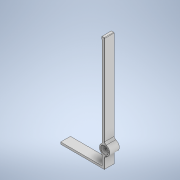
# Autodesk Inventor part: Fan PDP Lid
Saved by Autodesk Inventor 2020.3 (Build 243373010, 373A)
## iProperties
Created: 2019-12-31
Part Number: Fan PDP Lid
Material: Generic
Document SubType Name: Modeling
Designer: pepd9
Density: 1 g/cm^3
Appearance: Default
Author: pepd9
Autodesk Inventor part; units mm, degrees
ref_plane "YZ Plane" through (0, 0, 0) normal (1, 0, 0) x (0, 1, 0)
ref_plane "XZ Plane" through (0, 0, 0) normal (0, 1, 0) x (-1, 0, 0)
ref_plane "XY Plane" through (0, 0, 0) normal (0, 0, 1) x (1, 0, 0)
sketch "Sketch1" plane through (0, 0, 0) normal (0, 0, 1) x (1, 0, 0)
  line L0 (17.1597, -40.1235) -> (17.1597, -50)
  line L1 (17.1597, -50) -> (19.1597, -50)
  line L2 (19.1597, -50) -> (19.1597, -41.1847)
  arc A0 (20.5443, -39.2817) -> (19.1597, -41.1847) centre (21.1597, -41.1847) ccw
  arc A1 (20.5443, -39.2817) -> (20.5443, -30.7183) centre (19.1597, -35) ccw
  arc A2 (19.1597, -28.8153) -> (20.5443, -30.7183) centre (21.1597, -28.8153) ccw
  line L3 (19.1597, -28.8153) -> (19.1597, 49.6)
  arc A3 (19.1597, 49.6) -> (18.7597, 50) centre (18.7597, 49.6) ccw
  line L4 (18.7597, 50) -> (16.7597, 50)
  arc A4 (17.1597, 47.6) -> (16.7597, 48) centre (16.7597, 47.6) ccw
  line L5 (17.1597, 47.6) -> (17.1597, -29.8765)
  arc A5 (16.3905, -31.453) -> (17.1597, -29.8765) centre (15.1597, -29.8765) ccw
  arc A6 (16.3905, -31.453) -> (16.3905, -38.547) centre (19.1597, -35) ccw
  arc A7 (17.1597, -40.1235) -> (16.3905, -38.547) centre (15.1597, -40.1235) ccw
  line L6 (-19.1597, -50) -> (19.1597, -50)
  line L7 (19.1597, -50) -> (19.1597, -48)
  line L8 (19.1597, -48) -> (-19.1597, -48)
  line L9 (-19.1597, -48) -> (-19.1597, -50)
  circle A8 centre (19.1597, -35) radius 2.2
  line L10 (16.7597, 50) -> (16.7597, 48)
  point P0 (0, 0)
  point P1 (17.1605, -50)
  point P2 (17.1597, -48)
  dimension "d0" = 2
  constraints: 22 end point, 16 point on circle, 9 centre point, 1 horizontal, 1 parallel, 1 point on line
  measures "d0" distance between parallel lines of L8 L6
extrude "Extrusion1" add sketch "Sketch1" along normal blind 7 contours A7 A6 A5 L5 A4 L10 L4 A3 L3 A2 A1 A0 L2 L8 L0 | L8 L2 L1 L0 | L0 L6 L9 L8 | A8
sketch "Sketch2" plane through (0, 0, 7) normal (0, 0, 1) x (1, 0, 0)
  line L0 (-19.1597, -50) -> (19.1597, -50) projected
  line L1 (19.1597, -50) -> (19.1597, -41.1847) projected
  arc A0 (20.5443, -39.2817) -> (19.1597, -41.1847) centre (21.1597, -41.1847) ccw projected
  arc A1 (20.5443, -39.2817) -> (20.5443, -30.7183) centre (19.1597, -35) ccw projected
  arc A2 (19.1597, -28.8153) -> (20.5443, -30.7183) centre (21.1597, -28.8153) ccw projected
  line L2 (19.1597, -28.8153) -> (19.1597, 49.6) projected
  arc A3 (19.1597, 49.6) -> (18.7597, 50) centre (18.7597, 49.6) ccw projected
  line L3 (18.7597, 50) -> (16.7597, 50) projected
  arc A4 (17.1597, 47.6) -> (16.7597, 48) centre (16.7597, 47.6) ccw projected
  line L4 (17.1597, 47.6) -> (17.1597, -29.8765) projected
  arc A5 (16.3905, -31.453) -> (17.1597, -29.8765) centre (15.1597, -29.8765) ccw projected
  arc A6 (16.3905, -31.453) -> (16.3905, -38.547) centre (19.1597, -35) ccw projected
  arc A7 (17.1597, -40.1235) -> (16.3905, -38.547) centre (15.1597, -40.1235) ccw projected
  line L5 (17.1597, -40.1235) -> (17.1597, -48) projected
  line L6 (17.1597, -48) -> (-19.1597, -48) projected
  line L7 (16.7597, 50) -> (16.7597, 48) projected
  line L8 (-19.1597, -48) -> (-19.1597, -50) projected
  point P0 (0, 0)
extrude "Extrusion2" add sketch "Sketch2" along normal blind 1.5
fillet "Fillet1" radius 0.4 2 edges at (19.1597, -50, 7.75) (19.1597, -50, 3.5)
sketch "Sketch3" plane through (0, 0, 8.5) normal (0, 0, 1) x (1, 0, 0)
  line L0 (-17.1597, -48) -> (-17.1597, 26.9323) projected
  line L1 (-19.1597, -50) -> (18.7597, -50) projected
  arc A0 (18.7597, -50) -> (19.1597, -49.6) centre (18.7597, -49.6) ccw projected
  line L2 (19.1597, -49.6) -> (19.1597, -41.1847) projected
  arc A1 (20.5443, -39.2817) -> (19.1597, -41.1847) centre (21.1597, -41.1847) ccw projected
  arc A2 (20.5443, -39.2817) -> (20.5443, -30.7183) centre (19.1597, -35) ccw projected
  arc A3 (19.1597, -28.8153) -> (20.5443, -30.7183) centre (21.1597, -28.8153) ccw projected
  line L3 (19.1597, -28.8153) -> (19.1597, 49.6) projected
  arc A4 (19.1597, 49.6) -> (18.7597, 50) centre (18.7597, 49.6) ccw projected
  line L4 (18.7597, 50) -> (16.7597, 50) projected
  line L5 (16.7597, 50) -> (16.7597, 48) projected
  arc A5 (17.1597, 47.6) -> (16.7597, 48) centre (16.7597, 47.6) ccw projected
  line L6 (17.1597, 47.6) -> (17.1597, -29.8765) projected
  arc A6 (16.3905, -31.453) -> (17.1597, -29.8765) centre (15.1597, -29.8765) ccw projected
  arc A7 (16.3905, -31.453) -> (16.3905, -38.547) centre (19.1597, -35) ccw projected
  arc A8 (17.1597, -40.1235) -> (16.3905, -38.547) centre (15.1597, -40.1235) ccw projected
  line L7 (17.1597, -40.1235) -> (17.1597, -48) projected
  line L8 (17.1597, -48) -> (-19.1597, -48) projected
  line L9 (-19.1597, -48) -> (-19.1597, -50) projected
  point P0 (0, 0)
  point P1 (-4.5248, -20.5041)
  point P2 (-13.7791, 32.7713)
  constraints: 1 other
hole "Hole1" at (19.1597, -35, 8.5) at (-13.7791, 32.7713, 8.5) direction (0, 0, -1) diameter 3.4 end through all counterbore diameter 6.5 counterbore depth 3 clearance for "Socket Head Cap Screw" size "M3" standard "Ansi Metric M Profile"
sketch "Sketch4" plane through (19.1597, -35, 5.5) normal (0, 0, 1) x (1, 0, 0)
  circle A0 centre (0, 0) radius 3.25 projected
  circle A1 centre (0, 0) radius 3.25 projected
  circle A2 centre (0, 0) radius 1.7 projected
  circle A3 centre (-32.9388, 67.7713) radius 3.25 projected
  circle A4 centre (-32.9388, 67.7713) radius 1.7 projected
  line L0 (6.1601, -1.7) -> (-6.1601, -1.7)
  line L1 (-6.1601, -1.7) -> (-6.1601, 1.7)
  line L2 (-6.1601, 1.7) -> (6.1601, 1.7)
  line L3 (6.1601, 1.7) -> (6.1601, -1.7)
  circle A5 centre (0, 0) radius 3.25 projected
  line L4 (6.1601, -1.7) -> (-6.1601, 1.7) construction
  line L5 (-6.1601, -1.7) -> (6.1601, 1.7) construction
  arc A6 (-35.3905, 72.9289) -> (-38.3194, 65.8579) centre (-28.3194, 65.8579) ccw projected
  line L6 (-28.2339, 66.0713) -> (-37.6437, 66.0713)
  line L7 (-37.6437, 66.0713) -> (-37.6437, 69.4713)
  line L8 (-37.6437, 69.4713) -> (-28.2339, 69.4713)
  line L9 (-28.2339, 69.4713) -> (-28.2339, 66.0713)
  circle A7 centre (-32.9388, 67.7713) radius 1.7 projected
  line L10 (-28.2339, 66.0713) -> (-37.6437, 69.4713) construction
  line L11 (-37.6437, 66.0713) -> (-28.2339, 69.4713) construction
  point P0 (-19.1597, 35)
  point P1 (-30.1689, 69.4713)
  point P2 (-32.9388, 69.4713)
  point P3 (-32.9388, 66.0713)
  point P4 (-30.1689, 66.0713)
  point P5 (-35.7087, 69.4713)
  point P6 (-35.7087, 66.0713)
  point P7 (0, 1.7)
  point P8 (-2.7699, 1.7)
  point P9 (-2.7699, -1.7)
  point P10 (0, -1.7)
  point P11 (2.7699, 1.7)
  point P12 (2.7699, -1.7)
  dimension "d13" = 3.4
  dimension "d14" = 3.4
  constraints: 24 end point, 4 midpoint, 4 parallel, 2 horizontal, 2 perpendicular, 1 point on circle
  measures "d13" distance of L0.end L1.end
  measures "d14" distance of L6.end L7.end
extrude "Extrusion3" cut sketch "Sketch4" against normal blind 0.5 contours A0 L0 A2 L2 | L2 A2 L0 A0 | A3 L6 A4 L8 | L8 A4 L6 A3
sketch "Sketch5" plane through (19.1597, -35, 5) normal (0, 0, 1) x (1, 0, 0)
  arc A0 (-32.9388, 69.4713) -> (-32.9388, 66.0713) centre (-32.9388, 67.7713) ccw projected
  line L0 (-35.7087, 69.4713) -> (-32.9388, 69.4713) projected
  arc A1 (-35.7087, 69.4713) -> (-35.7087, 66.0713) centre (-32.9388, 67.7713) ccw projected
  line L1 (-32.9388, 66.0713) -> (-35.7087, 66.0713) projected
  arc A2 (-30.1689, 66.0713) -> (-30.1689, 69.4713) centre (-32.9388, 67.7713) ccw projected
  line L2 (-32.9388, 69.4713) -> (-30.1689, 69.4713) projected
  arc A3 (-32.9388, 66.0713) -> (-32.9388, 69.4713) centre (-32.9388, 67.7713) ccw projected
  line L3 (-30.1689, 66.0713) -> (-32.9388, 66.0713) projected
  arc A4 (0, 1.7) -> (0, -1.7) centre (0, 0) ccw projected
  line L4 (-2.7699, 1.7) -> (0, 1.7) projected
  arc A5 (-2.7699, 1.7) -> (-2.7699, -1.7) centre (0, 0) ccw projected
  line L5 (0, -1.7) -> (-2.7699, -1.7) projected
  line L6 (2.7699, -1.7) -> (0, -1.7) projected
  arc A6 (2.7699, -1.7) -> (2.7699, 1.7) centre (0, 0) ccw projected
  line L7 (0, 1.7) -> (2.7699, 1.7) projected
  arc A7 (0, -1.7) -> (0, 1.7) centre (0, 0) ccw projected
  line L8 (1.7, 1.7) -> (-1.7, 1.7)
  line L9 (-1.7, 1.7) -> (-1.7, -1.7)
  line L10 (-1.7, -1.7) -> (1.7, -1.7)
  line L11 (1.7, -1.7) -> (1.7, 1.7)
  line L12 (1.7, 1.7) -> (-1.7, -1.7) construction
  line L13 (-1.7, 1.7) -> (1.7, -1.7) construction
  line L14 (-31.2388, 66.0713) -> (-34.6388, 66.0713)
  line L15 (-34.6388, 66.0713) -> (-34.6388, 69.4713)
  line L16 (-34.6388, 69.4713) -> (-31.2388, 69.4713)
  line L17 (-31.2388, 69.4713) -> (-31.2388, 66.0713)
  line L18 (-31.2388, 66.0713) -> (-34.6388, 69.4713) construction
  line L19 (-34.6388, 66.0713) -> (-31.2388, 69.4713) construction
  point P0 (-19.1597, 35)
  point P1 (1.7, -1.7)
  point P2 (1.7, 1.7)
  point P3 (-1.7, 1.7)
  point P4 (-1.7, -1.7)
  dimension "d17" = 3.4
  dimension "d18" = 3.4
  dimension "d19" = 3.4
  dimension "d20" = 3.4
  constraints: 24 end point, 4 midpoint, 4 parallel, 2 horizontal, 2 perpendicular
  measures "d17" distance of L10.end L9.end
  measures "d18" distance of L9.end L8.end
  measures "d19" distance of L15.end L16.end
  measures "d20" distance of L14.end L15.end
extrude "Extrusion4" cut sketch "Sketch5" against normal blind 0.5 contours A3 A0 | A0 L15 L0 | L2 L17 A3 | A0 L1 L15 | L17 L3 A3 | A7 A4 | A4 L9 L4 | L7 L11 A7 | A4 L5 L9 | L11 L6 A7
sketch "Sketch6" plane through (0, 0, 8.5) normal (0, 0, 1) x (1, 0, 0)
  line L0 (-17.2523, -48.0084) -> (-17.2523, -4.1232) construction
  line L1 (-17.2523, -4.1232) -> (-6.8496, -4.1232) construction
  line L2 (-6.8496, -4.1232) -> (-6.8496, -48.0084) construction
  line L3 (-6.8496, -48.0084) -> (-17.2523, -48.0084) construction
  line L4 (-6.9988, -47.4715) -> (-16.9988, -47.4715)
  line L5 (-16.9988, -47.4715) -> (-16.9988, -43.5714)
  spline S0 degree 2 poles (-16.9988, -43.5714) (-16.9988, -42.2142) (-15.8131, -40.8048) (-14.5379, -40.596) knots 0 0 0 1 2 2 2
  spline S1 degree 2 poles (-14.5379, -40.596) (-14.1203, -40.5364) (-13.8295, -40.5214) (-13.7176, -40.5214) knots 0 0 0 1 2 2 2
  spline S2 degree 2 poles (-13.7176, -40.5214) (-12.3082, -40.5214) (-10.7273, -42.2664) (-10.7273, -43.825) knots 0 0 0 1 2 2 2
  line L6 (-10.7273, -43.825) -> (-10.7273, -44.6154)
  line L7 (-10.7273, -44.6154) -> (-6.9988, -44.6154)
  line L8 (-6.9988, -44.6154) -> (-6.9988, -47.4715)
  spline S3 degree 2 poles (-12.8302, -44.1904) (-12.8302, -43.9816) (-13.1807, -43.5341) (-13.5387, -43.4596) knots 0 0 0 1 2 2 2
  spline S4 degree 2 poles (-13.5387, -43.4596) (-13.7251, -43.4223) (-13.8892, -43.4223) knots 0 0 0 1 1 1
  spline S5 degree 2 poles (-13.8892, -43.4223) (-14.3515, -43.4223) (-14.8809, -43.8548) (-14.8809, -44.1605) knots 0 0 0 1 2 2 2
  line L9 (-14.8809, -44.1605) -> (-14.8809, -44.6154)
  line L10 (-14.8809, -44.6154) -> (-12.8302, -44.6154)
  line L11 (-12.8302, -44.6154) -> (-12.8302, -44.1904)
  line L12 (-6.9988, -40.1188) -> (-16.9988, -40.1188)
  line L13 (-16.9988, -40.1188) -> (-16.9988, -34.1083)
  line L14 (-16.9988, -34.1083) -> (-14.6871, -34.1083)
  line L15 (-14.6871, -34.1083) -> (-14.6871, -37.2627)
  line L16 (-14.6871, -37.2627) -> (-13.1956, -37.2627)
  line L17 (-13.1956, -37.2627) -> (-13.1956, -34.3022)
  line L18 (-13.1956, -34.3022) -> (-10.9809, -34.3022)
  line L19 (-10.9809, -34.3022) -> (-10.9809, -37.2627)
  line L20 (-10.9809, -37.2627) -> (-9.3105, -37.2627)
  line L21 (-9.3105, -37.2627) -> (-9.3105, -34.0039)
  line L22 (-9.3105, -34.0039) -> (-6.9988, -34.0039)
  line L23 (-6.9988, -34.0039) -> (-6.9988, -40.1188)
  line L24 (-6.9988, -33.3552) -> (-16.9988, -33.3552)
  line L25 (-16.9988, -33.3552) -> (-16.9988, -29.4551)
  spline S6 degree 2 poles (-16.9988, -29.4551) (-16.9988, -28.0979) (-15.8131, -26.6885) (-14.5379, -26.4797) knots 0 0 0 1 2 2 2
  spline S7 degree 2 poles (-14.5379, -26.4797) (-14.1203, -26.42) (-13.8295, -26.4051) (-13.7176, -26.4051) knots 0 0 0 1 2 2 2
  spline S8 degree 2 poles (-13.7176, -26.4051) (-12.3082, -26.4051) (-10.7273, -28.1501) (-10.7273, -29.7086) knots 0 0 0 1 2 2 2
  line L26 (-10.7273, -29.7086) -> (-10.7273, -30.4991)
  line L27 (-10.7273, -30.4991) -> (-6.9988, -30.4991)
  line L28 (-6.9988, -30.4991) -> (-6.9988, -33.3552)
  spline S9 degree 2 poles (-12.8302, -30.074) (-12.8302, -29.8652) (-13.1807, -29.4178) (-13.5387, -29.3432) knots 0 0 0 1 2 2 2
  spline S10 degree 2 poles (-13.5387, -29.3432) (-13.7251, -29.3059) (-13.8892, -29.3059) knots 0 0 0 1 1 1
  spline S11 degree 2 poles (-13.8892, -29.3059) (-14.3515, -29.3059) (-14.8809, -29.7384) (-14.8809, -30.0442) knots 0 0 0 1 2 2 2
  line L29 (-14.8809, -30.0442) -> (-14.8809, -30.4991)
  line L30 (-14.8809, -30.4991) -> (-12.8302, -30.4991)
  line L31 (-12.8302, -30.4991) -> (-12.8302, -30.074)
  line L32 (-13.2255, -15.3835) -> (-13.2255, -18.1352)
  line L33 (-13.2255, -18.1352) -> (-13.8892, -18.1426)
  spline S12 degree 2 poles (-13.8892, -18.1426) (-14.3813, -18.1426) (-14.7169, -18.1948) (-15.0226, -18.3216) (-15.1718, -18.5751) (-15.1718, -18.7392) knots 0 0 0 1 2 3 4 4 4
  spline S13 degree 2 poles (-15.1718, -18.7392) (-15.1718, -18.9331) (-14.866, -19.2388) (-13.8817, -19.3134) (-11.8235, -19.3134) knots 0 0 0 1 2 3 3 3
  spline S14 degree 2 poles (-11.8235, -19.3134) (-10.2202, -19.3134) (-9.2807, -19.2388) (-9.0868, -19.1419) knots 0 0 0 1 2 2 2
  spline S15 degree 2 poles (-9.0868, -19.1419) (-8.781, -18.9853) (-8.781, -18.6572) knots 0 0 0 1 1 1
  spline S16 degree 2 poles (-8.781, -18.6572) (-8.781, -18.4558) (-9.0868, -18.1501) (-9.7057, -18.0457) (-10.7199, -18.0457) knots 0 0 0 1 2 3 3 3
  line L34 (-10.7199, -18.0457) -> (-11.1673, -18.0457)
  line L35 (-11.1673, -18.0457) -> (-11.1673, -15.2567)
  spline S17 degree 2 poles (-11.1673, -15.2567) (-10.8839, -15.2567) (-10.6006, -15.2567) (-10.4514, -15.2567) knots 0 0 0 1 2 2 2
  spline S18 degree 2 poles (-10.4514, -15.2567) (-8.6319, -15.2567) (-6.8496, -16.9495) (-6.8496, -18.7168) knots 0 0 0 1 2 2 2
  spline S19 degree 2 poles (-6.8496, -18.7168) (-6.8496, -19.0822) (-6.8944, -19.4849) knots 0 0 0 1 1 1
  spline S20 degree 2 poles (-6.8944, -19.4849) (-7.0211, -20.9465) (-8.0204, -21.5654) knots 0 0 0 1 1 1
  spline S21 degree 2 poles (-8.0204, -21.5654) (-9.0495, -22.1993) (-11.391, -22.1993) knots 0 0 0 1 1 1
  line L36 (-11.391, -22.1993) -> (-11.7937, -22.2366)
  line L37 (-11.7937, -22.2366) -> (-11.9876, -22.2366)
  line L38 (-11.9876, -22.2366) -> (-13.5387, -22.1993)
  spline S22 degree 2 poles (-13.5387, -22.1993) (-15.224, -22.1993) (-16.9242, -20.7899) (-17.0883, -19.2985) knots 0 0 0 1 2 2 2
  spline S23 degree 2 poles (-17.0883, -19.2985) (-17.133, -18.8212) (-17.133, -18.4484) knots 0 0 0 1 1 1
  spline S24 degree 2 poles (-17.133, -18.4484) (-17.133, -16.8525) (-15.4328, -15.3835) (-13.6282, -15.3835) knots 0 0 0 1 2 2 2
  line L39 (-13.6282, -15.3835) -> (-13.2255, -15.3835)
  spline S25 degree 2 poles (-12.2038, -14.9286) (-14.3291, -14.9286) (-15.6043, -14.2053) knots 0 0 0 1 1 1
  spline S26 degree 2 poles (-15.6043, -14.2053) (-17.2523, -13.2806) (-17.2523, -11.3194) knots 0 0 0 1 1 1
  spline S27 degree 2 poles (-17.2523, -11.3194) (-17.2523, -10.7079) (-17.0584, -9.895) (-16.872, -9.5669) knots 0 0 0 1 2 2 2
  spline S28 degree 2 poles (-16.872, -9.5669) (-16.35, -8.4931) (-14.4335, -7.7325) (-12.2038, -7.7325) knots 0 0 0 1 2 2 2
  spline S29 degree 2 poles (-12.2038, -7.7325) (-9.3776, -7.7325) (-6.8795, -9.0151) (-6.8795, -10.5438) knots 0 0 0 1 2 2 2
  spline S30 degree 2 poles (-6.8795, -10.5438) (-6.8795, -12.4752) (-7.476, -13.4894) knots 0 0 0 1 1 1
  spline S31 degree 2 poles (-7.476, -13.4894) (-8.0055, -14.3842) (-9.0644, -14.7049) knots 0 0 0 1 1 1
  spline S32 degree 2 poles (-9.0644, -14.7049) (-9.7952, -14.9286) (-11.1748, -14.9286) knots 0 0 0 1 1 1
  spline S33 degree 2 poles (-11.1748, -14.9286) (-11.4208, -14.9286) (-11.9279, -14.9286) (-12.2038, -14.9286) knots 0 0 0 1 2 2 2
  spline S34 degree 2 poles (-11.309, -12.0054) (-9.6908, -12.0054) (-8.7959, -11.7071) (-8.7959, -11.3194) knots 0 0 0 1 2 2 2
  spline S35 degree 2 poles (-8.7959, -11.3194) (-8.7959, -10.954) (-9.6833, -10.6557) (-11.309, -10.6557) knots 0 0 0 1 2 2 2
  line L40 (-11.309, -10.6557) -> (-12.7408, -10.6557)
  spline S36 degree 2 poles (-12.7408, -10.6557) (-14.3217, -10.6557) (-15.2165, -10.954) (-15.2165, -11.3194) knots 0 0 0 1 2 2 2
  spline S37 degree 2 poles (-15.2165, -11.3194) (-15.2165, -11.6922) (-14.3291, -12.0054) (-12.7408, -12.0054) knots 0 0 0 1 2 2 2
  line L41 (-12.7408, -12.0054) -> (-11.309, -12.0054)
  line L42 (-6.9988, -7.0241) -> (-9.6982, -7.0241)
  line L43 (-9.6982, -7.0241) -> (-9.6982, -4.4141)
  line L44 (-9.6982, -4.4141) -> (-6.9988, -4.4141)
  line L45 (-6.9988, -4.4141) -> (-6.9988, -7.0241)
  point P0 (0, 0)
  constraints: 2 other
extrude "Extrusion5" cut sketch "Sketch6" against normal blind 0.6
sketch "Sketch7" plane through (0, 0, 8.5) normal (0, 0, 1) x (1, 0, 0)
  line L0 (-3.7937, -33.6465) -> (-3.7937, -2.887) construction
  line L1 (-3.7937, -2.887) -> (-12.6472, -2.887) construction
  line L2 (-12.6472, -2.887) -> (-12.6472, -33.6465) construction
  line L3 (-12.6472, -33.6465) -> (-3.7937, -33.6465) construction
  line L4 (3.9744, -28.2269) -> (3.9744, 29.3109) construction
  line L5 (3.9744, 29.3109) -> (-4.8792, 29.3109) construction
  line L6 (-4.8792, 29.3109) -> (-4.8792, -28.2269) construction
  line L7 (-4.8792, -28.2269) -> (3.9744, -28.2269) construction
  line L8 (-3.7937, -31.8232) -> (-1.4209, -32.0663)
  line L9 (-1.4209, -32.0663) -> (-1.4209, -32.8929)
  line L10 (-1.4209, -32.8929) -> (-3.7937, -33.136)
  line L11 (-3.7937, -33.136) -> (-3.7937, -31.8232)
  line L12 (-3.7937, -30.1263) -> (-1.4209, -30.3694)
  line L13 (-1.4209, -30.3694) -> (-1.4209, -31.196)
  line L14 (-1.4209, -31.196) -> (-3.7937, -31.4391)
  line L15 (-3.7937, -31.4391) -> (-3.7937, -30.1263)
  line L16 (2.4737, -27.8362) -> (-2.3837, -27.8362)
  line L17 (-2.3837, -27.8362) -> (-2.3837, -29.6109)
  line L18 (-2.3837, -29.6109) -> (-3.5263, -29.6109)
  line L19 (-3.5263, -29.6109) -> (-3.5263, -24.5541)
  line L20 (-3.5263, -24.5541) -> (-2.3837, -24.5541)
  line L21 (-2.3837, -24.5541) -> (-2.3837, -26.3289)
  line L22 (-2.3837, -26.3289) -> (2.4737, -26.3289)
  line L23 (2.4737, -26.3289) -> (2.4737, -27.8362)
  line L24 (2.4737, -23.9366) -> (-3.5263, -23.9366)
  line L25 (-3.5263, -23.9366) -> (-3.5263, -19.8815)
  line L26 (-3.5263, -19.8815) -> (-2.3837, -19.8815)
  line L27 (-2.3837, -19.8815) -> (-2.3837, -22.4391)
  line L28 (-2.3837, -22.4391) -> (-1.3285, -22.4391)
  line L29 (-1.3285, -22.4391) -> (-1.3285, -20.0809)
  line L30 (-1.3285, -20.0809) -> (-0.1859, -20.0809)
  line L31 (-0.1859, -20.0809) -> (-0.1859, -22.4391)
  line L32 (-0.1859, -22.4391) -> (1.3311, -22.4391)
  line L33 (1.3311, -22.4391) -> (1.3311, -19.8815)
  line L34 (1.3311, -19.8815) -> (2.4737, -19.8815)
  line L35 (2.4737, -19.8815) -> (2.4737, -23.9366)
  line L36 (2.4737, -12.734) -> (2.4737, -14.2316)
  line L37 (2.4737, -14.2316) -> (-1.5036, -14.2316)
  line L38 (-1.5036, -14.2316) -> (1.0637, -15.3208)
  line L39 (1.0637, -15.3208) -> (1.0637, -16.3515)
  line L40 (1.0637, -16.3515) -> (-1.5036, -17.4407)
  line L41 (-1.5036, -17.4407) -> (2.4737, -17.4407)
  line L42 (2.4737, -17.4407) -> (2.4737, -18.8605)
  line L43 (2.4737, -18.8605) -> (-3.5263, -18.8605)
  line L44 (-3.5263, -18.8605) -> (-3.5263, -17.1246)
  line L45 (-3.5263, -17.1246) -> (-0.5652, -15.7924)
  line L46 (-0.5652, -15.7924) -> (-3.5263, -14.4699)
  line L47 (-3.5263, -14.4699) -> (-3.5263, -12.734)
  line L48 (-3.5263, -12.734) -> (2.4737, -12.734)
  spline S0 degree 2 poles (-1.6349, -6.875) (-1.2167, -6.875) (-0.4582, -7.1425) (-0.2054, -7.3904) knots 0 0 0 1 2 2 2
  spline S1 degree 2 poles (-0.2054, -7.3904) (-0.0449, -7.5412) (0.2176, -7.9107) (0.31, -8.1295) knots 0 0 0 1 2 2 2
  spline S2 degree 2 poles (0.31, -8.1295) (0.4024, -8.3532) (0.5094, -8.8734) (0.5094, -9.1943) knots 0 0 0 1 2 2 2
  line L49 (0.5094, -9.1943) -> (0.5094, -9.982)
  line L50 (0.5094, -9.982) -> (2.4737, -9.982)
  line L51 (2.4737, -9.982) -> (2.4737, -11.4893)
  line L52 (2.4737, -11.4893) -> (-3.5263, -11.4893)
  line L53 (-3.5263, -11.4893) -> (-3.5263, -9.1603)
  spline S3 degree 2 poles (-3.5263, -9.1603) (-3.5263, -8.6449) (-3.3367, -7.8913) (-3.1324, -7.5849) knots 0 0 0 1 2 2 2
  spline S4 degree 2 poles (-3.1324, -7.5849) (-2.9039, -7.2446) (-2.1551, -6.875) (-1.6349, -6.875) knots 0 0 0 1 2 2 2
  spline S5 degree 2 poles (-1.596, -8.4212) (-1.8537, -8.4212) (-2.2183, -8.6644) (-2.2864, -8.8297) knots 0 0 0 1 2 2 2
  spline S6 degree 2 poles (-2.2864, -8.8297) (-2.3788, -9.0436) (-2.408, -9.4326) (-2.408, -9.7681) knots 0 0 0 1 2 2 2
  line L54 (-2.408, -9.7681) -> (-2.408, -9.982)
  line L55 (-2.408, -9.982) -> (-0.6089, -9.982)
  line L56 (-0.6089, -9.982) -> (-0.6089, -9.875)
  spline S7 degree 2 poles (-0.6089, -9.875) (-0.6089, -9.666) (-0.6187, -9.2867) (-0.643, -9.1457) knots 0 0 0 1 2 2 2
  spline S8 degree 2 poles (-0.643, -9.1457) (-0.6624, -9.0242) (-0.7791, -8.7567) (-0.852, -8.6838) knots 0 0 0 1 2 2 2
  spline S9 degree 2 poles (-0.852, -8.6838) (-0.9979, -8.5282) (-1.3237, -8.4212) (-1.596, -8.4212) knots 0 0 0 1 2 2 2
  spline S10 degree 2 poles (-0.5263, -0.6076) (0.9324, -0.6076) (2.6001, -2.1635) (2.6001, -3.5152) knots 0 0 0 1 2 2 2
  spline S11 degree 2 poles (2.6001, -3.5152) (2.6001, -4.8718) (0.9129, -6.418) (-0.5263, -6.418) knots 0 0 0 1 2 2 2
  spline S12 degree 2 poles (-0.5263, -6.418) (-1.9704, -6.418) (-3.6527, -4.8718) (-3.6527, -3.5152) knots 0 0 0 1 2 2 2
  spline S13 degree 2 poles (-3.6527, -3.5152) (-3.6527, -2.1635) (-1.9801, -0.6076) (-0.5263, -0.6076) knots 0 0 0 1 2 2 2
  spline S14 degree 2 poles (-0.5263, -2.1635) (-1.066, -2.1635) (-1.8196, -2.3823) (-2.0579, -2.572) knots 0 0 0 1 2 2 2
  spline S15 degree 2 poles (-2.0579, -2.572) (-2.3059, -2.7616) (-2.5198, -3.2478) (-2.5198, -3.5104) knots 0 0 0 1 2 2 2
  spline S16 degree 2 poles (-2.5198, -3.5104) (-2.5198, -3.7875) (-2.3204, -4.2397) (-2.0676, -4.4488) knots 0 0 0 1 2 2 2
  spline S17 degree 2 poles (-2.0676, -4.4488) (-1.8342, -4.6336) (-1.0611, -4.8621) (-0.5263, -4.8621) knots 0 0 0 1 2 2 2
  spline S18 degree 2 poles (-0.5263, -4.8621) (0.028, -4.8621) (0.7574, -4.6433) (1.0053, -4.4537) knots 0 0 0 1 2 2 2
  spline S19 degree 2 poles (1.0053, -4.4537) (1.2533, -4.264) (1.4672, -3.7729) (1.4672, -3.5104) knots 0 0 0 1 2 2 2
  spline S20 degree 2 poles (1.4672, -3.5104) (1.4672, -3.243) (1.2387, -2.747) (0.9956, -2.5671) knots 0 0 0 1 2 2 2
  spline S21 degree 2 poles (0.9956, -2.5671) (0.733, -2.3726) (0.0377, -2.1635) (-0.5263, -2.1635) knots 0 0 0 1 2 2 2
  line L57 (2.4737, 5.83) -> (2.4737, 3.9969)
  line L58 (2.4737, 3.9969) -> (0.2711, 2.3292)
  line L59 (0.2711, 2.3292) -> (0.2711, 1.7846)
  line L60 (0.2711, 1.7846) -> (2.4737, 1.7846)
  line L61 (2.4737, 1.7846) -> (2.4737, 0.287)
  line L62 (2.4737, 0.287) -> (-3.5263, 0.287)
  line L63 (-3.5263, 0.287) -> (-3.5263, 2.6987)
  spline S22 degree 2 poles (-3.5263, 2.6987) (-3.5263, 3.1995) (-3.3999, 3.9386) (-3.2054, 4.2546) knots 0 0 0 1 2 2 2
  spline S23 degree 2 poles (-3.2054, 4.2546) (-3.0012, 4.5755) (-2.3642, 4.9548) (-1.878, 4.9548) knots 0 0 0 1 2 2 2
  spline S24 degree 2 poles (-1.878, 4.9548) (-1.1924, 4.9548) (-0.3318, 4.3324) (-0.079, 3.8121) knots 0 0 0 1 2 2 2
  line L64 (-0.079, 3.8121) -> (2.4737, 5.83)
  spline S25 degree 2 poles (-1.6884, 3.4086) (-1.9169, 3.4086) (-2.2426, 3.2335) (-2.3302, 3.0342) knots 0 0 0 1 2 2 2
  spline S26 degree 2 poles (-2.3302, 3.0342) (-2.3885, 2.8932) (-2.4226, 2.548) (-2.4226, 2.2903) knots 0 0 0 1 2 2 2
  line L65 (-2.4226, 2.2903) -> (-2.4226, 1.7846)
  line L66 (-2.4226, 1.7846) -> (-0.8083, 1.7846)
  line L67 (-0.8083, 1.7846) -> (-0.8083, 2.2173)
  spline S27 degree 2 poles (-0.8083, 2.2173) (-0.8083, 2.5285) (-0.8861, 2.971) (-1.0076, 3.1217) knots 0 0 0 1 2 2 2
  spline S28 degree 2 poles (-1.0076, 3.1217) (-1.1243, 3.2676) (-1.4355, 3.4086) (-1.6884, 3.4086) knots 0 0 0 1 2 2 2
  line L68 (2.4737, 5.6306) -> (-3.5263, 7.6582)
  line L69 (-3.5263, 7.6582) -> (-3.5263, 9.3016)
  line L70 (-3.5263, 9.3016) -> (2.4737, 11.3292)
  line L71 (2.4737, 11.3292) -> (2.4737, 9.7781)
  line L72 (2.4737, 9.7781) -> (1.2484, 9.4037)
  line L73 (1.2484, 9.4037) -> (1.2484, 7.5172)
  line L74 (1.2484, 7.5172) -> (2.4737, 7.1379)
  line L75 (2.4737, 7.1379) -> (2.4737, 5.6306)
  line L76 (0.1593, 9.0731) -> (-1.8245, 8.4604)
  line L77 (-1.8245, 8.4604) -> (0.1593, 7.8429)
  line L78 (0.1593, 7.8429) -> (0.1593, 9.0731)
  line L79 (2.4737, 17.4702) -> (2.4737, 15.6371)
  line L80 (2.4737, 15.6371) -> (0.2711, 13.9694)
  line L81 (0.2711, 13.9694) -> (0.2711, 13.4248)
  line L82 (0.2711, 13.4248) -> (2.4737, 13.4248)
  line L83 (2.4737, 13.4248) -> (2.4737, 11.9272)
  line L84 (2.4737, 11.9272) -> (-3.5263, 11.9272)
  line L85 (-3.5263, 11.9272) -> (-3.5263, 14.3389)
  spline S29 degree 2 poles (-3.5263, 14.3389) (-3.5263, 14.8397) (-3.3999, 15.5788) (-3.2054, 15.8948) knots 0 0 0 1 2 2 2
  spline S30 degree 2 poles (-3.2054, 15.8948) (-3.0012, 16.2157) (-2.3642, 16.595) (-1.878, 16.595) knots 0 0 0 1 2 2 2
  spline S31 degree 2 poles (-1.878, 16.595) (-1.1924, 16.595) (-0.3318, 15.9726) (-0.079, 15.4523) knots 0 0 0 1 2 2 2
  line L86 (-0.079, 15.4523) -> (2.4737, 17.4702)
  spline S32 degree 2 poles (-1.6884, 15.0488) (-1.9169, 15.0488) (-2.2426, 14.8737) (-2.3302, 14.6744) knots 0 0 0 1 2 2 2
  spline S33 degree 2 poles (-2.3302, 14.6744) (-2.3885, 14.5334) (-2.4226, 14.1882) (-2.4226, 13.9305) knots 0 0 0 1 2 2 2
  line L87 (-2.4226, 13.9305) -> (-2.4226, 13.4248)
  line L88 (-2.4226, 13.4248) -> (-0.8083, 13.4248)
  line L89 (-0.8083, 13.4248) -> (-0.8083, 13.8575)
  spline S34 degree 2 poles (-0.8083, 13.8575) (-0.8083, 14.1687) (-0.8861, 14.6112) (-1.0076, 14.7619) knots 0 0 0 1 2 2 2
  spline S35 degree 2 poles (-1.0076, 14.7619) (-1.1243, 14.9078) (-1.4355, 15.0488) (-1.6884, 15.0488) knots 0 0 0 1 2 2 2
  line L90 (-3.5263, 22.9062) -> (-0.0303, 20.8348)
  line L91 (-0.0303, 20.8348) -> (2.4737, 20.8348)
  line L92 (2.4737, 20.8348) -> (2.4737, 19.3275)
  line L93 (2.4737, 19.3275) -> (0.0426, 19.3275)
  line L94 (0.0426, 19.3275) -> (-3.5263, 17.2222)
  line L95 (-3.5263, 17.2222) -> (-3.5263, 18.9386)
  line L96 (-3.5263, 18.9386) -> (-1.3869, 20.1104)
  line L97 (-1.3869, 20.1104) -> (-3.5263, 21.2433)
  line L98 (-3.5263, 21.2433) -> (-3.5263, 22.9062)
  line L99 (-3.7937, 24.6517) -> (-1.4209, 24.4086)
  line L100 (-1.4209, 24.4086) -> (-1.4209, 23.582)
  line L101 (-1.4209, 23.582) -> (-3.7937, 23.3389)
  line L102 (-3.7937, 23.3389) -> (-3.7937, 24.6517)
  line L103 (-3.7937, 26.3486) -> (-1.4209, 26.1055)
  line L104 (-1.4209, 26.1055) -> (-1.4209, 25.2789)
  line L105 (-1.4209, 25.2789) -> (-3.7937, 25.0358)
  line L106 (-3.7937, 25.0358) -> (-3.7937, 26.3486)
  spline S36 degree 2 poles (7.9419, -23.3453) (8.4136, -23.3453) (9.211, -23.6662) (9.4979, -23.9822) knots 0 0 0 1 2 2 2
  spline S37 degree 2 poles (9.4979, -23.9822) (9.7847, -24.2983) (10.1008, -25.1637) (10.1008, -25.7958) knots 0 0 0 1 2 2 2
  spline S38 degree 2 poles (10.1008, -25.7958) (10.0959, -26.4668) (9.8771, -27.4295) (9.7361, -27.7456) knots 0 0 0 1 2 2 2
  line L107 (9.7361, -27.7456) -> (8.4282, -27.7456)
  line L108 (8.4282, -27.7456) -> (8.4282, -27.6094)
  spline S39 degree 2 poles (8.4282, -27.6094) (8.4914, -27.4928) (8.6567, -27.2107) (8.7442, -26.9822) knots 0 0 0 1 2 2 2
  spline S40 degree 2 poles (8.7442, -26.9822) (8.8269, -26.7683) (8.9387, -26.3258) (8.9387, -26.0584) knots 0 0 0 1 2 2 2
  spline S41 degree 2 poles (8.9387, -26.0584) (8.9387, -25.825) (8.822, -25.2804) (8.6664, -25.1151) knots 0 0 0 1 2 2 2
  spline S42 degree 2 poles (8.6664, -25.1151) (8.5449, -24.9936) (8.2483, -24.8574) (8.0003, -24.8574) knots 0 0 0 1 2 2 2
  spline S43 degree 2 poles (8.0003, -24.8574) (7.7863, -24.8574) (7.4849, -25.0325) (7.3925, -25.1735) knots 0 0 0 1 2 2 2
  spline S44 degree 2 poles (7.3925, -25.1735) (7.2564, -25.3777) (7.1786, -25.9611) (7.1786, -26.1702) knots 0 0 0 1 2 2 2
  spline S45 degree 2 poles (7.1786, -26.1702) (7.1786, -26.5009) (7.2855, -27.1281) (7.3439, -27.3566) knots 0 0 0 1 2 2 2
  line L109 (7.3439, -27.3566) -> (7.3439, -27.4879)
  line L110 (7.3439, -27.4879) -> (3.9744, -27.4879)
  line L111 (3.9744, -27.4879) -> (3.9744, -23.5106)
  line L112 (3.9744, -23.5106) -> (5.1073, -23.5106)
  line L113 (5.1073, -23.5106) -> (5.1073, -26.0633)
  line L114 (5.1073, -26.0633) -> (6.104, -26.0633)
  spline S46 degree 2 poles (6.104, -26.0633) (6.0943, -25.9417) (6.0846, -25.6062) (6.0846, -25.5138) knots 0 0 0 1 2 2 2
  spline S47 degree 2 poles (6.0846, -25.5138) (6.0846, -25.0811) (6.2596, -24.3517) (6.4395, -24.0649) knots 0 0 0 1 2 2 2
  spline S48 degree 2 poles (6.4395, -24.0649) (6.6632, -23.7245) (7.4071, -23.3453) (7.9419, -23.3453) knots 0 0 0 1 2 2 2
  line L115 (3.9744, -17.3404) -> (9.9744, -19.402)
  line L116 (9.9744, -19.402) -> (9.9744, -20.9725)
  line L117 (9.9744, -20.9725) -> (3.9744, -23.0341)
  line L118 (3.9744, -23.0341) -> (3.9744, -21.4733)
  line L119 (3.9744, -21.4733) -> (8.044, -20.1654)
  line L120 (8.044, -20.1654) -> (3.9744, -18.8623)
  line L121 (3.9744, -18.8623) -> (3.9744, -17.3404)
  line L122 (5.117, -10.3485) -> (5.117, -12.8671)
  line L123 (5.117, -12.8671) -> (6.2499, -12.8671)
  line L124 (6.2499, -12.8671) -> (6.2499, -10.5479)
  line L125 (6.2499, -10.5479) -> (7.3925, -10.5479)
  line L126 (7.3925, -10.5479) -> (7.3925, -12.8671)
  line L127 (7.3925, -12.8671) -> (9.9744, -12.8671)
  line L128 (9.9744, -12.8671) -> (9.9744, -14.3647)
  line L129 (9.9744, -14.3647) -> (3.9744, -14.3647)
  line L130 (3.9744, -14.3647) -> (3.9744, -10.3485)
  line L131 (3.9744, -10.3485) -> (5.117, -10.3485)
  line L132 (9.9744, -10.2172) -> (3.9744, -8.1897)
  line L133 (3.9744, -8.1897) -> (3.9744, -6.5462)
  line L134 (3.9744, -6.5462) -> (9.9744, -4.5187)
  line L135 (9.9744, -4.5187) -> (9.9744, -6.0697)
  line L136 (9.9744, -6.0697) -> (8.7491, -6.4441)
  line L137 (8.7491, -6.4441) -> (8.7491, -8.3307)
  line L138 (8.7491, -8.3307) -> (9.9744, -8.7099)
  line L139 (9.9744, -8.7099) -> (9.9744, -10.2172)
  line L140 (7.6599, -6.7748) -> (5.6761, -7.3874)
  line L141 (5.6761, -7.3874) -> (7.6599, -8.0049)
  line L142 (7.6599, -8.0049) -> (7.6599, -6.7748)
  line L143 (9.9744, 1.2188) -> (9.9744, -0.2302)
  line L144 (9.9744, -0.2302) -> (5.7928, -2.5446)
  line L145 (5.7928, -2.5446) -> (9.9744, -2.5446)
  line L146 (9.9744, -2.5446) -> (9.9744, -3.9206)
  line L147 (9.9744, -3.9206) -> (3.9744, -3.9206)
  line L148 (3.9744, -3.9206) -> (3.9744, -2.073)
  line L149 (3.9744, -2.073) -> (7.412, -0.1573)
  line L150 (7.412, -0.1573) -> (3.9744, -0.1573)
  line L151 (3.9744, -0.1573) -> (3.9744, 1.2188)
  line L152 (3.9744, 1.2188) -> (9.9744, 1.2188)
  spline S49 degree 2 poles (5.8658, 9.47) (6.2839, 9.47) (7.0424, 9.2025) (7.2953, 8.9546) knots 0 0 0 1 2 2 2
  spline S50 degree 2 poles (7.2953, 8.9546) (7.4557, 8.8038) (7.7183, 8.4343) (7.8107, 8.2155) knots 0 0 0 1 2 2 2
  spline S51 degree 2 poles (7.8107, 8.2155) (7.903, 7.9919) (8.01, 7.4716) (8.01, 7.1507) knots 0 0 0 1 2 2 2
  line L153 (8.01, 7.1507) -> (8.01, 6.363)
  line L154 (8.01, 6.363) -> (9.9744, 6.363)
  line L155 (9.9744, 6.363) -> (9.9744, 4.8557)
  line L156 (9.9744, 4.8557) -> (3.9744, 4.8557)
  line L157 (3.9744, 4.8557) -> (3.9744, 7.1847)
  spline S52 degree 2 poles (3.9744, 7.1847) (3.9744, 7.7001) (4.164, 8.4538) (4.3682, 8.7601) knots 0 0 0 1 2 2 2
  spline S53 degree 2 poles (4.3682, 8.7601) (4.5967, 9.1004) (5.3455, 9.47) (5.8658, 9.47) knots 0 0 0 1 2 2 2
  spline S54 degree 2 poles (5.9047, 7.9238) (5.647, 7.9238) (5.2823, 7.6807) (5.2142, 7.5154) knots 0 0 0 1 2 2 2
  spline S55 degree 2 poles (5.2142, 7.5154) (5.1218, 7.3014) (5.0927, 6.9124) (5.0927, 6.5769) knots 0 0 0 1 2 2 2
  line L158 (5.0927, 6.5769) -> (5.0927, 6.363)
  line L159 (5.0927, 6.363) -> (6.8917, 6.363)
  line L160 (6.8917, 6.363) -> (6.8917, 6.47)
  spline S56 degree 2 poles (6.8917, 6.47) (6.8917, 6.679) (6.882, 7.0583) (6.8577, 7.1993) knots 0 0 0 1 2 2 2
  spline S57 degree 2 poles (6.8577, 7.1993) (6.8382, 7.3209) (6.7215, 7.5883) (6.6486, 7.6612) knots 0 0 0 1 2 2 2
  spline S58 degree 2 poles (6.6486, 7.6612) (6.5027, 7.8168) (6.1769, 7.9238) (5.9047, 7.9238) knots 0 0 0 1 2 2 2
  spline S59 degree 2 poles (6.9792, 15.6304) (7.8204, 15.6304) (9.1429, 14.8962) (9.4979, 14.3371) knots 0 0 0 1 2 2 2
  spline S60 degree 2 poles (9.4979, 14.3371) (9.7993, 13.8703) (9.9744, 12.7714) (9.9744, 12.1539) knots 0 0 0 1 2 2 2
  line L161 (9.9744, 12.1539) -> (9.9744, 10.2771)
  line L162 (9.9744, 10.2771) -> (3.9744, 10.2771)
  line L163 (3.9744, 10.2771) -> (3.9744, 12.1345)
  spline S61 degree 2 poles (3.9744, 12.1345) (3.9744, 12.7666) (4.1348, 13.8703) (4.446, 14.3565) knots 0 0 0 1 2 2 2
  spline S62 degree 2 poles (4.446, 14.3565) (4.8252, 14.9449) (6.1089, 15.6304) (6.9792, 15.6304) knots 0 0 0 1 2 2 2
  spline S63 degree 2 poles (6.9695, 14.0842) (6.3763, 14.0842) (5.5303, 13.6758) (5.292, 13.2577) knots 0 0 0 1 2 2 2
  spline S64 degree 2 poles (5.292, 13.2577) (5.1267, 12.9513) (5.0927, 12.2803) (5.0927, 11.8136) knots 0 0 0 1 2 2 2
  line L164 (5.0927, 11.8136) -> (5.0927, 11.7844)
  line L165 (5.0927, 11.7844) -> (8.8512, 11.7844)
  line L166 (8.8512, 11.7844) -> (8.8512, 11.8136)
  spline S65 degree 2 poles (8.8512, 11.8136) (8.8512, 12.3192) (8.8171, 13.0145) (8.6178, 13.3306) knots 0 0 0 1 2 2 2
  spline S66 degree 2 poles (8.6178, 13.3306) (8.3844, 13.7001) (7.5627, 14.0842) (6.9695, 14.0842) knots 0 0 0 1 2 2 2
  spline S67 degree 2 poles (5.8658, 21.1393) (6.2839, 21.1393) (7.0424, 20.8719) (7.2953, 20.6239) knots 0 0 0 1 2 2 2
  spline S68 degree 2 poles (7.2953, 20.6239) (7.4557, 20.4732) (7.7183, 20.1037) (7.8107, 19.8849) knots 0 0 0 1 2 2 2
  spline S69 degree 2 poles (7.8107, 19.8849) (7.903, 19.6612) (8.01, 19.141) (8.01, 18.8201) knots 0 0 0 1 2 2 2
  line L167 (8.01, 18.8201) -> (8.01, 18.0324)
  line L168 (8.01, 18.0324) -> (9.9744, 18.0324)
  line L169 (9.9744, 18.0324) -> (9.9744, 16.5251)
  line L170 (9.9744, 16.5251) -> (3.9744, 16.5251)
  line L171 (3.9744, 16.5251) -> (3.9744, 18.8541)
  spline S70 degree 2 poles (3.9744, 18.8541) (3.9744, 19.3695) (4.164, 20.1231) (4.3682, 20.4295) knots 0 0 0 1 2 2 2
  spline S71 degree 2 poles (4.3682, 20.4295) (4.5967, 20.7698) (5.3455, 21.1393) (5.8658, 21.1393) knots 0 0 0 1 2 2 2
  spline S72 degree 2 poles (5.9047, 19.5931) (5.647, 19.5931) (5.2823, 19.35) (5.2142, 19.1847) knots 0 0 0 1 2 2 2
  spline S73 degree 2 poles (5.2142, 19.1847) (5.1218, 18.9708) (5.0927, 18.5818) (5.0927, 18.2463) knots 0 0 0 1 2 2 2
  line L172 (5.0927, 18.2463) -> (5.0927, 18.0324)
  line L173 (5.0927, 18.0324) -> (6.8917, 18.0324)
  line L174 (6.8917, 18.0324) -> (6.8917, 18.1393)
  spline S74 degree 2 poles (6.8917, 18.1393) (6.8917, 18.3484) (6.882, 18.7277) (6.8577, 18.8687) knots 0 0 0 1 2 2 2
  spline S75 degree 2 poles (6.8577, 18.8687) (6.8382, 18.9902) (6.7215, 19.2577) (6.6486, 19.3306) knots 0 0 0 1 2 2 2
  spline S76 degree 2 poles (6.6486, 19.3306) (6.5027, 19.4862) (6.1769, 19.5931) (5.9047, 19.5931) knots 0 0 0 1 2 2 2
  point P0 (0, 0)
  constraints: 4 other
extrude "Extrusion6" cut sketch "Sketch7" against normal blind 0.6
chamfer "Chamfer1" distance 0.25 angle 45 10 edges at (-0.2, -50, 8.5) (19.0425, -49.8828, 8.5) (19.1597, -45.3923, 8.5) (19.5425, -40.008, 8.5) (23.6597, -35, 8.5) (19.5425, -29.992, 8.5) (19.1597, 10.3923, 8.5) (19.0425, 49.8828, 8.5) (17.7597, 50, 8.5) (19.1597, -31.75, 8.5)
fillet "Fillet2" radius 0.4 1 edges at (17.1597, -48, 4.25)
body "Solid1"
